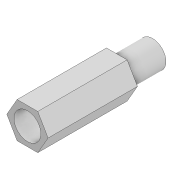
# Autodesk Inventor part: piedino
Saved by Autodesk Inventor 2022 (Build 260153000, 153)
## iProperties
Created: 2025-08-17
Part Number: piedino
Material: Generic
Document SubType Name: Modeling
Designer: sacchie
Density: 1 g/cm^3
Appearance: Default
Author: sacchie
Autodesk Inventor part; units mm, degrees
ref_plane "YZ Plane" through (0, 0, 0) normal (1, 0, 0) x (0, 1, 0)
ref_plane "XZ Plane" through (0, 0, 0) normal (0, 1, 0) x (-1, 0, 0)
ref_plane "XY Plane" through (0, 0, 0) normal (0, 0, 1) x (1, 0, 0)
sketch "Sketch1" plane through (0, 0, 0) normal (0, 0, 1) x (1, 0, 0)
  circle A0 centre (0, 0) radius 1.5
  dimension "d0" = 3
  constraints: 1 centre point, 1 coincident
  measures "d0" diameter of A0
extrude "Extrusion1" add sketch "Sketch1" along normal blind 4
sketch "Sketch2" plane through (0, 0, 4) normal (0, 0, 1) x (1, 0, 0)
  circle A0 centre (0, 0) radius 1.5 construction
  line L0 (0.866, 1.5) -> (1.7321, 0) construction
  line L1 (1.7321, 0) -> (0.866, -1.5)
  line L2 (0.866, -1.5) -> (-0.866, -1.5)
  line L3 (-0.866, -1.5) -> (-1.7321, 0)
  line L4 (-1.7321, 0) -> (-0.866, 1.5)
  line L5 (-0.866, 1.5) -> (0.866, 1.5)
  line L6 (2.3094, 0) -> (1.1547, 2)
  line L7 (1.1547, 2) -> (-1.1547, 2)
  line L8 (-1.1547, 2) -> (-2.3094, 0)
  line L9 (-2.3094, 0) -> (-1.1547, -2)
  line L10 (-1.1547, -2) -> (1.1547, -2)
  line L11 (1.1547, -2) -> (2.3094, 0)
  point P0 (0, 1.5)
  dimension "d3" = 0.5
  constraints: 24 end point, 1 coincident, 1 midpoint, 1 vertical alignment, 19 other
  measures "d3" distance between parallel lines of L0 L6
extrude "Extrusion2" add sketch "Sketch2" along normal blind 10
sketch "Sketch3" plane through (0, 0, 14) normal (0, 0, 1) x (1, 0, 0)
  circle A0 centre (0, 0) radius 1.5
  dimension "d6" = 3
  constraints: 1 centre point, 1 coincident
  measures "d6" diameter of A0
extrude "Extrusion3" cut sketch "Sketch3" against normal blind 4
body "Solid1"
